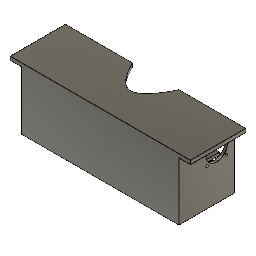
casing_redisgn v2 (Autodesk Fusion 360 design; units mm, degrees)
Autodesk Fusion 360 part; units mm, degrees
sketch "Sketch1" plane through (0, 0, 0) normal (0, 1, 0) x (1, 0, 0)
  line L0 (-85, -35) -> (85, -35)
  line L1 (85, -35) -> (85, 31)
  line L2 (85, 31) -> (-85, 31)
  line L3 (-85, 31) -> (-85, -35)
  dimension "d1" = 170
  dimension "d2" = 66
  constraint horizontal L0
  constraint vertical L1
  constraint horizontal L2
  constraint vertical L3
  measures "d1" distance of L0.start L0.end
  measures "d2" distance of L0.start L2.end
extrude "Extrude1" add sketch "Sketch1" along normal blind 3 makes body 1
extrude "Extrude2" add sketch "Sketch1" along normal blind 60 thin wall 3 inside bodies 1
sketch "Sketch2" plane through (0, 0, 35) normal (0, 0, 1) x (-1, 0, 0)
  line L0 (85, 0) -> (-85, 0)
  line L1 (-85, 0) -> (-85, -60)
  line L2 (-85, -60) -> (85, -60)
  line L3 (85, -60) -> (85, 0)
  line L4 (-97.5, 0) -> (97.5, 0)
  line L5 (97.5, 0) -> (97.5, -60)
  line L6 (97.5, -60) -> (-97.5, -60)
  line L7 (-97.5, -60) -> (-97.5, 0)
  dimension "d8" = 195
  dimension "d9" = 60
  constraint horizontal L4
  constraint vertical L5
  constraint horizontal L6
  constraint vertical L7
  measures "d8" distance of L4.start L4.end
  measures "d9" distance of L4.start L6.end
extrude "Extrude3" add sketch "Sketch2" along normal blind -3 and the other way blind -1 bodies 1
sketch "Sketch4" plane through (0, 60, 0) normal (0, 1, 0) x (-1, 0, 0)
  line L0 (82, 32) -> (82, -28)
  line L1 (82, -28) -> (-82, -28)
  line L2 (-82, -28) -> (-82, 32)
  line L3 (-82, 32) -> (82, 32)
  line L4 (85, 32) -> (97.5, 32)
  line L5 (97.5, 32) -> (97.5, 36)
  line L6 (97.5, 36) -> (-97.5, 36)
  line L7 (-97.5, 36) -> (-97.5, 32)
  line L8 (-97.5, 32) -> (-85, 32)
  line L9 (-85, 32) -> (-85, -31)
  line L10 (-85, -31) -> (85, -31)
  line L11 (85, -31) -> (85, 32)
  circle A0 centre (-75, 30) radius 3
  circle A1 centre (75, 30) radius 3
  line L12 (-72, 30) -> (-72, 32)
  line L13 (-78, 30) -> (-78, 32)
  line L14 (-78, 32) -> (-72, 32)
  line L15 (78, 30) -> (78, 32)
  line L16 (72, 30) -> (72, 32)
  line L17 (72, 32) -> (78, 32)
  circle A2 centre (0, -26) radius 3
  line L18 (3, -26.0059) -> (2.9961, -28)
  line L19 (-3, -26.0059) -> (-2.9961, -28)
  line L20 (-2.9961, -28) -> (2.9961, -28)
  dimension "d51" = 6
  constraint coincident A0 L12.start
  constraint coincident L3 L12.end
  constraint tangent A0 L12
  constraint perpendicular L3 L12
  constraint coincident A0 L13.start
  constraint coincident L3 L13.end
  constraint tangent A0 L13
  constraint perpendicular L3 L13
  constraint coincident A1 L15.start
  constraint coincident L3 L15.end
  constraint tangent A1 L15
  constraint perpendicular L3 L15
  constraint coincident A1 L16.start
  constraint coincident L3 L16.end
  constraint tangent A1 L16
  constraint perpendicular L3 L16
  constraint coincident A2 L18.start
  constraint coincident L1 L18.end
  constraint tangent A2 L18
  constraint coincident A2 L19.start
  constraint coincident L1 L19.end
  constraint tangent A2 L19
  measures "d51" diameter of A2
extrude "Extrude4" add sketch "Sketch4" against normal blind 4 contours L3 A1 L15 L17 | L1 A2 L18 L20 | L3 A1 L17 | L1 A2 L20 | L1 A2 L20 | L3 A1 L16 L17 | L1 A2 L19 L20 | L3 A0 L12 L14 | L3 A0 L14 | L3 A0 L13 L14 picked at (74.0546, 30.2743) picked at (-75.9454, 30.2743) bodies 1
fillet "Fillet1" radius 2.5 4 edges at (-78, 58, 32) (-72, 58, 32) (78, 58, 32) (72, 58, 32) on bodies 1
cylinder "CylinderPrimitive1" add diameter 25 height 35 placed x (1, 0, 0) y (0, 1, 0) z (0, 0, 1) at (43.2918, 39.8377, -28) separate body makes body 2
move_face "MoveFace1" to x (1, 0, 0) y (0, 1, 0) z (0, 0, 1) at (25, 0, 0) 1 faces at (55.7297, 38.5931, -16.3333) on bodies 2
pattern_linear "R-Pattern1" count 6 spacing 26 along (-1, 0, 0) of bodies 2 makes body 3 at (54.7297, 38.5931, -16.3333) makes body 4 at (28.7297, 38.5931, -16.3333) makes body 5 at (2.7297, 38.5931, -16.3333) makes body 6 at (-23.2703, 38.5931, -16.3333) makes body 7 at (-49.2703, 38.5931, -16.3333)
move_face "MoveFace2" to x (1, 0, 0) y (0, 1, 0) z (0, 0, 1) at (-7, 0, 0) 3 faces at (2.7297, 38.5931, -16.3333) (-23.2703, 38.5931, -16.3333) (-49.2703, 38.5931, -16.3333) on bodies 5 6 7
move_face "MoveFace3" to x (1, 0, 0) y (0, 1, 0) z (0, 0, 1) at (0.208, 0, 0) 3 faces at (80.7297, 38.5931, -16.3333) (54.7297, 38.5931, -16.3333) (28.7297, 38.5931, -16.3333) on bodies 2 3 4
move_face "MoveFace4" to x (1, 0, 0) y (0, 1, 0) z (0, 0, 1) at (0.208, 0, 0) 3 faces at (-56.2703, 38.5931, -16.3333) (-30.2703, 38.5931, -16.3333) (-4.2703, 38.5931, -16.3333) on bodies 5 6 7
sketch "Sketch6" plane through (0, 3, 0) normal (0, 1, 0) x (-1, 0, 0)
  line L0 (-82, -28) -> (82, -28)
  line L1 (82, -28) -> (82, 32)
  line L2 (82, 32) -> (-82, 32)
  line L3 (-82, 32) -> (-82, -28)
  circle A0 centre (-76, 26) radius 1.5
  circle A1 centre (-76, 26) radius 3
  circle A2 centre (76, 26) radius 1.5
  circle A3 centre (76, 26) radius 3
  circle A4 centre (-76, -22) radius 1.5
  circle A5 centre (-76, -22) radius 3
  circle A6 centre (76, -22) radius 1.5
  circle A7 centre (76, -22) radius 3
  dimension "d35" = 3
  dimension "d36" = 6
  dimension "d39" = 152
  dimension "d40" = -48
  constraint concentric A0 A1
  measures "d35" diameter of A0
  measures "d36" diameter of A1
extrude "Extrude5" add sketch "Sketch6" along normal blind 3 contours A0 | A1 bodies 1
hole "Hole1" at (76, 6, 26) direction (0, -1, 0) diameter 2.529 depth 3 tip angle 180 bodies 1
thread "Thread1" "ISO Metric profile 3.0 M3x0.5 6H" major diameter 3.086 minor diameter 2.529 pitch 0.5 angle 60 resizes the face on face at (76.4325, 5, 24.8118) on bodies 1
extrude "Extrude6" add sketch "Sketch6" along normal blind 3 contours A2 | A3 | A4 | A5 | A6 | A7 bodies 1
hole "Hole2" at (-76, 3, -22) at (-76, 3, 26) at (76, 3, -22) direction (0, 1, 0) diameter 2.529 depth 3 tip angle 180 bodies 1
thread "Thread2" "ISO Metric profile 3.0 M3x0.5 6H" major diameter 3.086 minor diameter 2.529 pitch 0.5 angle 60 resizes the face on face at (-75.5675, 4, 27.1882) on face at (-75.5675, 4, -20.8118) on face at (76.2506, 4, -23.2394) on bodies 1
fillet "Fillet2" radius 2.5 2 edges at (-2.9961, 58, -28) (2.9961, 58, -28) on bodies 1
hole "Hole3" at (75, 60, 30) direction (0, -1, 0) diameter 2.529 depth 3 tip angle 180 bodies 1
thread "Thread3" "ISO Metric profile 3.0 M3x0.5 6H"
hole "Hole4" at (0, 60, -26) direction (0, -1, 0) diameter 2.529 depth 3 tip angle 180 bodies 1
thread "Thread4" "ISO Metric profile 3.0 M3x0.5 6H"
hole "Hole5" at (-75, 60, 30) direction (0, -1, 0) diameter 2.529 depth 3 tip angle 180 bodies 1
thread "Thread5" "ISO Metric profile 3.0 M3x0.5 6H"
sketch "Panel" plane through (0, 3, 0) normal (0, 1, 0) x (-1, 0, 0)
  circle A0 centre (76, -22) radius 3
  circle A1 centre (76, 26) radius 3
  circle A2 centre (-76, -22) radius 3
  circle A3 centre (-76, 26) radius 3
  line L0 (-82, -28) -> (82, -28)
  line L1 (82, -28) -> (82, 32)
  line L2 (82, 32) -> (-82, 32)
  line L3 (-82, 32) -> (-82, -28)
  line L4 (143.4373, 18.8566) -> (305.4373, 18.8566)
  line L5 (305.4373, 18.8566) -> (305.4373, -39.1434)
  line L6 (305.4373, -39.1434) -> (143.4373, -39.1434)
  line L7 (143.4373, -39.1434) -> (143.4373, 18.8566)
  dimension "d63" = 162
  dimension "d64" = 58
  constraint horizontal L4
  constraint vertical L5
  constraint horizontal L6
  constraint vertical L7
  measures "d63" distance of L4.start L4.end
  measures "d64" distance of L4.start L6.end
extrude "Extrude7" add sketch "Panel" along normal blind 3 separate body contours L4 L5 L6 L7 makes body 8
sketch "Panel screw holes" plane through (0, 6, 0) normal (0, 1, 0) x (-1, 0, 0)
  line L0 (143.4373, -39.1434) -> (305.4373, -39.1434)
  line L1 (305.4373, -39.1434) -> (305.4373, 18.8566)
  line L2 (305.4373, 18.8566) -> (143.4373, 18.8566)
  line L3 (143.4373, 18.8566) -> (143.4373, -39.1434)
  circle A0 centre (300.9372, 14) radius 1.5
  circle A1 centre (148.9372, 14) radius 1.5
  circle A2 centre (300.9372, -34) radius 1.5
  circle A3 centre (148.9372, -34) radius 1.5
  dimension "d67" = 3
  dimension "d70" = -152
  dimension "d71" = -48
  measures "d67" diameter of A0
move_body "Move2" bodies 8 to x (1, 0, 0) y (0, 1, 0) z (0, 0, 1) at (-0.5, 0, 0)
hole "Hole6" at (-148.9372, 6, 14) at (-300.9372, 6, 14) at (-300.9372, 6, -34) at (-148.9372, 6, -34) direction (0, -1, 0) diameter 2.529 depth 3 tip angle 180 bodies 8
thread "Thread6" "ISO Metric profile 3.0 M3x0.5 6H" major diameter 3.086 minor diameter 2.529 pitch 0.5 angle 60 resizes the face on face at (-301.2492, 5, 15.2254) on face at (-149.8853, 5, 14.8367) on face at (-301.2492, 5, -32.7746) on face at (-149.8853, 5, -33.1633) on bodies 8
move_body "Move3" bodies 8 to x (1, 0, 0) y (0, 1, 0) z (0, 0, 1) at (225, 0, 12)
move_body "Move4" bodies 8 to x (1, 0, 0) y (0, 1, 0) z (0, 0, 1) at (0, 7, 0)
move_body "Move5" bodies 8 to x (1, 0, 0) y (0, 1, 0) z (0, 0, 1) at (-0.63, 0, 0)
sketch "Nose gap" plane through (0, 0, 36) normal (0, 0, 1) x (-1, 0, 0)
  line L0 (-97.5, -60) -> (97.5, -60)
  line L1 (97.5, -60) -> (97.5, 0)
  line L2 (97.5, 0) -> (-97.5, 0)
  line L3 (-97.5, 0) -> (-97.5, -60)
  line L4 (-25, -60) -> (25, -60)
  line L5 (0, -60) -> (0, -33)
  spline S0 degree 5 poles (-25, -60) (-24, -57.9521) (-22, -54.0352) (-19, -48.6963) (-15, -42.6686) (-10, -37.0753) (-5, -33.597) (0, -32.4061) (5, -33.597) (10, -37.0753) (15, -42.6686) (19, -48.6963) (22, -54.0352) (24, -57.9521) (25, -60) knots 0 0 0 0 0 0 0.1 0.2 0.3 0.4 0.5 0.6 0.7 0.8 0.9 1 1 1 1 1 1
  dimension "d75" = 50
  dimension "d76" = 27
  constraint coincident L0 L4.start
  constraint midpoint L4 L5.start
  constraint perpendicular L4 L5
  measures "d75" distance of L4.start L4.end
  measures "d76" distance of L5.start L5.end
extrude "Extrude8" cut sketch "Nose gap" against normal blind 4 contours L0 L4 L5 S0 | L0 L4 L5 S0 bodies 1
move_body "Move6" bodies 8 to x (1, 0, 0) y (0, 1, 0) z (0, 0, 1) at (0.567, 0, 0)
sketch "Shelf" plane through (0, 13, 0) normal (0, 1, 0) x (-1, 0, 0)
  circle A0 centre (76.0002, -22) radius 1.2645
  circle A1 centre (-75.9998, 26) radius 1.2645
  circle A2 centre (76.0002, 26) radius 1.2645
  circle A3 centre (-75.9998, -22) radius 1.2645
  line L0 (-80.9997, -27.1434) -> (81.0003, -27.1434)
  line L1 (81.0003, -27.1434) -> (81.0003, 30.8566)
  line L2 (81.0003, 30.8566) -> (-80.9997, 30.8566)
  line L3 (-80.9997, 30.8566) -> (-80.9997, -27.1434)
  line L4 (-80.9997, 8.5) -> (81.0003, 8.5)
  line L5 (81.0003, 8.5) -> (81.0003, 11.5)
  line L6 (81.0003, 11.5) -> (-80.9997, 11.5)
  line L7 (-80.9997, 11.5) -> (-80.9997, 8.5)
  dimension "d79" = 3
  constraint horizontal L4
  constraint vertical L5
  constraint horizontal L6
  constraint vertical L7
  constraint coincident L1 L5.end
  constraint coincident L3 L4.start
  measures "d79" distance of L4.start L6.end
extrude "Extrude9" add sketch "Shelf" along normal blind 35 contours L1 L3 L4 L5 L6 L7 bodies 8
sketch "Atomizer holes" plane through (0, 0, 11.5) normal (0, 0, 1) x (-1, 0, 0)
  line L0 (81.0003, -13) -> (-80.9997, -13)
  line L1 (-80.9997, -13) -> (-80.9997, -48)
  line L2 (-80.9997, -48) -> (81.0003, -48)
  line L3 (81.0003, -48) -> (81.0003, -13)
  circle A0 centre (-69.4997, -35.0285) radius 7
  circle A1 centre (-43.4997, -35.0285) radius 7
  circle A2 centre (-17.4995, -35.0285) radius 7
  circle A3 centre (17.5005, -35.0285) radius 7
  circle A4 centre (43.5005, -35.0285) radius 7
  circle A5 centre (69.5005, -35.0285) radius 7
  dimension "d83" = 14
  dimension "d84" = 26
  dimension "d86" = 14
  dimension "d88" = 14
  dimension "d89" = 35
  dimension "d90" = 14
  dimension "d91" = 26
  dimension "d92" = 14
  dimension "d93" = 26
  dimension "d94" = 14
  measures "d83" diameter of A0
  measures "d84" distance of A0.centre A1.centre
  measures "d86" diameter of A1
  measures "d88" diameter of A2
  measures "d89" distance of A2.centre A3.centre
  measures "d90" diameter of A3
  measures "d91" distance of A3.centre A4.centre
  measures "d92" diameter of A4
  measures "d93" distance of A4.centre A5.centre
  measures "d94" diameter of A5
move_face "MoveFace5" to x (1, 0, 0) y (0, 1, 0) z (0, 0, 1) at (1, 0, 0) 1 faces at (80.9377, 38.5931, -16.3333) on bodies 2
move_face "MoveFace6" to x (1, 0, 0) y (0, 1, 0) z (0, 0, 1) at (1, 0, 0) 1 faces at (54.9377, 38.5931, -16.3333) on bodies 3
move_face "MoveFace7" to x (1, 0, 0) y (0, 1, 0) z (0, 0, 1) at (1, 0, 0) 1 faces at (28.9377, 38.5931, -16.3333) on bodies 4
move_face "MoveFace8" to x (1, 0, 0) y (0, 1, 0) z (0, 0, 1) at (-1, 0, 0) 2 faces at (-56.0623, 38.5931, -16.3333) (-24.3778, 3, -5.7052) on bodies 1 7
move_face "MoveFace9" to x (1, 0, 0) y (0, 1, 0) z (0, 0, 1) at (-1, 0, 0) 1 faces at (-30.0623, 38.5931, -16.3333) on bodies 6
move_face "MoveFace10" to x (1, 0, 0) y (0, 1, 0) z (0, 0, 1) at (-1, 0, 0) 1 faces at (-4.0623, 38.5931, -16.3333) on bodies 5
extrude "Extrude10" cut sketch "Atomizer holes" against normal blind 3 contours A0 | A1 | A2 | A3 | A4 | A5 bodies 8
sketch "Fan" plane through (-85, 0, 0) normal (-1, 0, 0) x (0, -1, 0)
  line L0 (0, 32) -> (-60, 32)
  line L1 (-60, 32) -> (-60, -31)
  line L2 (-60, -31) -> (0, -31)
  line L3 (0, -31) -> (0, 32)
  line L4 (-53.3427, 32.1089) -> (-28.3427, 32.1089)
  line L5 (-28.3427, 32.1089) -> (-28.3427, 7.1089)
  line L6 (-28.3427, 7.1089) -> (-53.3427, 7.1089)
  line L7 (-53.3427, 7.1089) -> (-53.3427, 32.1089)
  line L8 (-53.3427, 32.1089) -> (-28.3427, 7.1089)
  line L9 (-53.3427, 7.1089) -> (-28.3427, 32.1089)
  circle A0 centre (-40.8427, 19.6089) radius 11.75
  circle A1 through (-29.0927, 19.6089, -170) (-46.7177, 29.7847, -170) (-46.7177, 9.4331, -170)
  line L10 (-53.3427, 32.1089) -> (-49.1512, 32.1089)
  line L11 (-49.1512, 32.1089) -> (-49.1512, 27.9174)
  line L12 (-49.1512, 27.9174) -> (-53.3427, 27.9174)
  line L13 (-53.3427, 27.9174) -> (-53.3427, 32.1089)
  line L14 (-28.3427, 32.1089) -> (-32.5342, 32.1089)
  line L15 (-32.5342, 32.1089) -> (-32.5342, 27.9174)
  line L16 (-32.5342, 27.9174) -> (-28.3427, 27.9174)
  line L17 (-28.3427, 27.9174) -> (-28.3427, 32.1089)
  line L18 (-28.3427, 7.1089) -> (-32.5342, 7.1089)
  line L19 (-32.5342, 7.1089) -> (-32.5342, 11.3004)
  line L20 (-32.5342, 11.3004) -> (-28.3427, 11.3004)
  line L21 (-28.3427, 11.3004) -> (-28.3427, 7.1089)
  line L22 (-53.3427, 7.1089) -> (-49.1512, 7.1089)
  line L23 (-49.1512, 7.1089) -> (-49.1512, 11.3004)
  line L24 (-49.1512, 11.3004) -> (-53.3427, 11.3004)
  line L25 (-53.3427, 11.3004) -> (-53.3427, 7.1089)
  line L26 (-49.1512, 32.1089) -> (-53.3427, 27.9174)
  line L27 (-32.5342, 32.1089) -> (-28.3427, 27.9174)
  line L28 (-32.5342, 7.1089) -> (-28.3427, 11.3004)
  line L29 (-49.1512, 7.1089) -> (-53.3427, 11.3004)
  circle A2 centre (-51.247, 30.0131) radius 1.4
  circle A3 centre (-51.247, 30.0131) radius 1.4
  circle A4 centre (-30.4385, 30.0131) radius 1.4
  circle A5 centre (-51.247, 9.2046) radius 1.4
  circle A6 centre (-30.4385, 9.2046) radius 1.4
  circle A7 through (-29.0385, 30.0131, -170) (-31.1385, 31.2256, -170) (-31.1385, 28.8007, -170)
  circle A8 through (-29.0385, 9.2046, -170) (-31.1385, 10.417, -170) (-31.1385, 7.9922, -170)
  circle A9 through (-49.847, 9.2046, -170) (-51.947, 10.417, -170) (-51.947, 7.9922, -170)
  circle A10 through (-49.847, 30.0131, -170) (-51.947, 31.2256, -170) (-51.947, 28.8007, -170)
  dimension "d97" = 25
  dimension "d98" = 25
  dimension "d99" = 23.5
  dimension "d102" = 23.5
  dimension "d105" = 2.8
  dimension "d106" = 2.8
  dimension "d107" = 2.8
  dimension "d108" = 2.8
  dimension "d109" = 2.8
  dimension "d113" = 2.8
  dimension "d114" = 2.8
  dimension "d115" = 2.8
  dimension "d116" = 2.8
  constraint horizontal L4
  constraint vertical L5
  constraint horizontal L6
  constraint vertical L7
  constraint midpoint L8 A0.centre
  constraint horizontal L10
  constraint vertical L11
  constraint horizontal L12
  constraint vertical L13
  constraint coincident A0 L11.end
  constraint coincident L8 L11.end
  constraint horizontal L14
  constraint vertical L15
  constraint horizontal L16
  constraint vertical L17
  constraint coincident L9 L15.end
  constraint coincident A0 L15.end
  constraint horizontal L18
  constraint vertical L19
  constraint horizontal L20
  constraint vertical L21
  constraint coincident L8 L19.end
  constraint coincident A0 L19.end
  constraint horizontal L22
  constraint vertical L23
  constraint horizontal L24
  constraint vertical L25
  constraint coincident L9 L23.end
  constraint coincident A0 L23.end
  constraint midpoint L26 A2.centre
  constraint midpoint L27 A4.centre
  constraint midpoint L29 A5.centre
  constraint midpoint L28 A6.centre
  measures "d97" distance of L4.start L4.end
  measures "d98" distance of L4.start L6.end
  measures "d99" diameter of A0
  measures "d105" diameter of A2
  measures "d106" diameter of A3
  measures "d107" diameter of A4
  measures "d108" diameter of A5
  measures "d109" diameter of A6
extrude "Extrude11" cut sketch "Fan" against normal blind 3 contours L8 L9 A0 | L8 L9 A0 | L8 L9 A0 | L8 L9 A0 bodies 1 7
extrude "Extrude12" cut sketch "Fan" along normal blind 3 contours A1 in plane through (85, 0, 0) normal (-1, 0, 0) bodies 1
hole "Hole7" at (-85, 51.247, 30.0131) at (-85, 30.4385, 30.0131) at (-85, 30.4385, 9.2046) at (-85, 51.247, 9.2046) direction (1, 0, 0) diameter 2.529 depth 3 tip angle 180 bodies 1
thread "Thread7" "ISO Metric profile 3.0 M3x0.5 6H" major diameter 3.086 minor diameter 2.529 pitch 0.5 angle 60 resizes the face on face at (-84, 51.3729, 7.9464) on face at (-84, 50.4835, 31.0211) on face at (-83, 30.5644, 10.4628) on face at (-83, 30.5644, 31.2713) on bodies 1
hole "Hole8" at (85, 30.4385, 30.0131) direction (-1, 0, 0) diameter 2.529 depth 3 tip angle 180 bodies 1
thread "Thread8" "ISO Metric profile 3.0 M3x0.5 6H" major diameter 3.086 minor diameter 2.529 pitch 0.5 angle 60 resizes the face on face at (83, 30.5644, 28.7549) on bodies 1
hole "Hole9" at (85, 51.247, 9.2046) direction (-1, 0, 0) diameter 2.529 depth 3 tip angle 180 bodies 1
thread "Thread9" "ISO Metric profile 3.0 M3x0.5 6H" major diameter 3.086 minor diameter 2.529 pitch 0.5 angle 60 resizes the face on face at (84, 51.3729, 10.4628) on bodies 1
hole "Hole10" at (85, 30.4385, 9.2046) direction (-1, 0, 0) diameter 2.529 depth 3 tip angle 180 bodies 1
thread "Thread10" "ISO Metric profile 3.0 M3x0.5 6H" major diameter 3.086 minor diameter 2.529 pitch 0.5 angle 60 resizes the face on face at (83, 30.5644, 7.9464) on bodies 1
hole "Hole11" at (85, 51.247, 30.0131) direction (-1, 0, 0) diameter 2.529 depth 3 tip angle 180 bodies 1
thread "Thread11" "ISO Metric profile 3.0 M3x0.5 6H" major diameter 3.086 minor diameter 2.529 pitch 0.5 angle 60 resizes the face on face at (84, 50.4835, 29.0051) on bodies 1
sketch "Spacer" plane through (0, 13, 0) normal (0, 1, 0) x (-1, 0, 0)
  line L0 (81.0003, 8.5) -> (-80.9997, 8.5)
  line L1 (-80.9997, 8.5) -> (-80.9997, -27.1434)
  line L2 (-80.9997, -27.1434) -> (81.0003, -27.1434)
  line L3 (81.0003, -27.1434) -> (81.0003, 8.5)
  circle A0 centre (-75.9998, -22) radius 1.2645
  circle A1 centre (76.0002, -22) radius 1.2645
  line L4 (-80.9997, -12.5184) -> (81.0003, -12.5184)
  line L5 (81.0003, -12.5184) -> (81.0003, -26.0184)
  line L6 (81.0003, -26.0184) -> (-80.9997, -26.0184)
  line L7 (-80.9997, -26.0184) -> (-80.9997, -12.5184)
  dimension "d129" = 162
  dimension "d130" = 13.5
  constraint horizontal L4
  constraint vertical L5
  constraint horizontal L6
  constraint vertical L7
  measures "d129" distance of L4.start L4.end
  measures "d130" distance of L4.start L6.end
extrude "Extrude13" add sketch "Spacer" along normal blind 8.65 separate body contours L1 L3 L4 L5 L6 L7 | A0 | A1 makes body 9
move_face "MoveFace11" to x (1, 0, 0) y (0, 1, 0) z (0, 0, 1) at (0, -5.5, 0) 6 faces at (81.9377, 38.5931, -16.3333) (55.9377, 38.5931, -16.3333) (29.9377, 38.5931, -16.3333) (-5.0623, 38.5931, -16.3333) (-31.0623, 38.5931, -16.3333) (-57.0623, 38.5931, -16.3333) on bodies 2 3 4 5 6 7
sketch "Sketch17" plane through (0, 13, 0) normal (0, 1, 0) x (-1, 0, 0)
  line L0 (81.0003, 8.5) -> (-80.9997, 8.5)
  line L1 (-80.9997, 8.5) -> (-80.9997, -27.1434)
  line L2 (-80.9997, -27.1434) -> (81.0003, -27.1434)
  line L3 (81.0003, -27.1434) -> (81.0003, 8.5)
  circle A0 centre (-75.9998, -22) radius 1.2645
  circle A1 centre (76.0002, -22) radius 1.2645
  line L4 (-78.6067, -27.1434) -> (-78.6067, -26.0184)
  line L5 (-78.6067, -26.0184) -> (-80.9997, -26.0184)
  line L6 (-78.6067, -26.0184) -> (81.0003, -26.0184)
  line L7 (-80.9997, -26.0184) -> (-80.9997, -12.5184)
  line L8 (-80.9997, -12.5184) -> (81.0003, -12.5184)
  line L9 (-80.9997, -16.4669) -> (-73.4997, -16.4669)
  line L10 (-73.4997, -12.5184) -> (-65.4997, -12.5184)
  line L11 (-65.4997, -12.5184) -> (-65.4997, -26.0184)
  line L12 (-65.4997, -26.0184) -> (-73.4997, -26.0184)
  line L13 (-73.4997, -26.0184) -> (-73.4997, -12.5184)
  line L14 (-65.4997, -12.5184) -> (-30.4997, -12.5184)
  line L15 (-65.4997, -12.5184) -> (-47.4997, -12.5184)
  line L16 (-47.4997, -12.5184) -> (-39.4997, -12.5184)
  line L17 (-39.4997, -12.5184) -> (-39.4997, -26.0184)
  line L18 (-39.4997, -26.0184) -> (-47.4997, -26.0184)
  line L19 (-47.4997, -26.0184) -> (-47.4997, -12.5184)
  line L20 (-39.4997, -12.5184) -> (-21.4997, -12.5184)
  line L21 (-21.4997, -12.5184) -> (-13.4997, -12.5184)
  line L22 (-13.4997, -12.5184) -> (-13.4997, -26.0184)
  line L23 (-13.4997, -26.0184) -> (-21.4997, -26.0184)
  line L24 (-21.4997, -26.0184) -> (-21.4997, -12.5184)
  line L25 (-13.4997, -12.5184) -> (13.5003, -12.5184)
  line L26 (13.5003, -12.5184) -> (21.5003, -12.5184)
  line L27 (21.5003, -12.5184) -> (21.5003, -26.0184)
  line L28 (21.5003, -26.0184) -> (13.5003, -26.0184)
  line L29 (13.5003, -26.0184) -> (13.5003, -12.5184)
  line L30 (21.5003, -12.5184) -> (39.5003, -12.5184)
  line L31 (39.5003, -12.5184) -> (47.5003, -12.5184)
  line L32 (47.5003, -12.5184) -> (47.5003, -26.0184)
  line L33 (47.5003, -26.0184) -> (39.5003, -26.0184)
  line L34 (39.5003, -26.0184) -> (39.5003, -12.5184)
  line L35 (47.5003, -12.5184) -> (65.5003, -12.5184)
  line L36 (65.5003, -12.5184) -> (73.5003, -12.5184)
  line L37 (73.5003, -12.5184) -> (73.5003, -26.0184)
  line L38 (73.5003, -26.0184) -> (65.5003, -26.0184)
  line L39 (65.5003, -26.0184) -> (65.5003, -12.5184)
  dimension "d133" = 1.125
  dimension "d134" = 13.5
  dimension "d135" = 162
  dimension "d136" = 7.5
  dimension "d137" = 8
  dimension "d138" = 35
  dimension "d139" = 18
  dimension "d140" = 8
  dimension "d141" = 13.5
  dimension "d142" = 18
  dimension "d143" = 8
  dimension "d144" = 13.5
  dimension "d145" = 27
  dimension "d146" = 8
  dimension "d147" = 13.5
  dimension "d148" = 18
  dimension "d149" = 8
  dimension "d150" = 13.5
  dimension "d151" = 18
  dimension "d152" = 8
  dimension "d153" = 13.5
  constraint coincident L2 L4.start
  constraint perpendicular L2 L4
  constraint coincident L1 L5.end
  constraint perpendicular L1 L5
  constraint coincident L3 L6.end
  constraint perpendicular L3 L6
  constraint perpendicular L5 L7
  constraint perpendicular L7 L8
  constraint coincident L7 L9.start
  constraint perpendicular L7 L9
  constraint horizontal L10
  constraint vertical L11
  constraint horizontal L12
  constraint vertical L13
  constraint coincident L8 L10.start
  constraint perpendicular L11 L14
  constraint perpendicular L11 L15
  constraint horizontal L16
  constraint vertical L17
  constraint horizontal L18
  constraint vertical L19
  constraint perpendicular L17 L20
  constraint horizontal L21
  constraint vertical L22
  constraint horizontal L23
  constraint vertical L24
  constraint perpendicular L22 L25
  constraint horizontal L26
  constraint vertical L27
  constraint horizontal L28
  constraint vertical L29
  constraint perpendicular L27 L30
  constraint horizontal L31
  constraint vertical L32
  constraint horizontal L33
  constraint vertical L34
  constraint perpendicular L32 L35
  constraint horizontal L36
  constraint vertical L37
  constraint horizontal L38
  constraint vertical L39
  measures "d133" distance of L4.start L4.end
  measures "d134" distance of L5.end L7.end
  measures "d135" distance of L7.end L8.end
  measures "d136" distance of L9.start L9.end
  measures "d137" distance of L10.start L10.end
  measures "d138" distance of L10.end L14.end
  measures "d139" distance of L10.end L15.end
  measures "d140" distance of L15.end L16.end
  measures "d141" distance of L15.end L18.end
  measures "d142" distance of L16.end L20.end
  measures "d143" distance of L20.end L21.end
  measures "d144" distance of L20.end L23.end
  measures "d145" distance of L21.end L25.end
  measures "d146" distance of L25.end L26.end
  measures "d147" distance of L25.end L28.end
  measures "d148" distance of L26.end L30.end
  measures "d149" distance of L30.end L31.end
  measures "d150" distance of L30.end L33.end
  measures "d151" distance of L31.end L35.end
  measures "d152" distance of L35.end L36.end
  measures "d153" distance of L35.end L38.end
extrude "Extrude14" cut sketch "Sketch17" against normal blind 3 contours L6 L8 L36 L37 L38 L39 | L6 L8 L10 L11 L12 L13 | L6 L8 L31 L32 L33 L34 | L6 L8 L14 L16 L17 L18 L19 | L6 L8 L26 L27 L28 L29 | L6 L8 L21 L22 L23 L24 bodies 8
hidden bodies 9
named bodies: "Housing", "Atomizer", "Atomizer (1)", "Atomizer (2)", "Atomizer (3)", "Atomizer (4)", "Atomizer (5)", "Inner panel", "Spacer"
